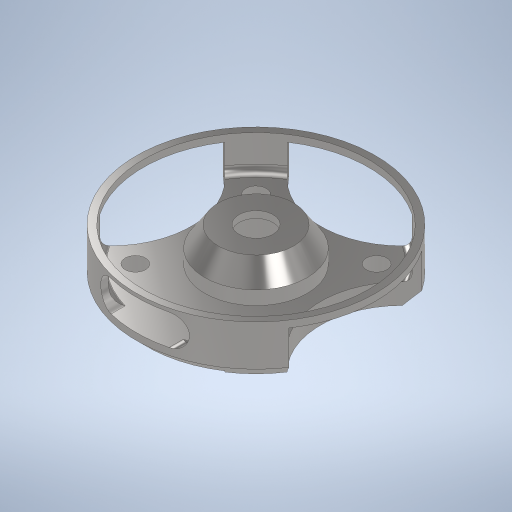
# Autodesk Inventor part: Base
Saved by Autodesk Inventor 2023.2 (Build 272271000, 271)
## iProperties
Created: 2023-03-04
Part Number: Base
Material: Stainless Steel
Document SubType Name: Modeling
Designer: Nathan Cai
Density: 8 g/cm^3
Appearance: Semi-Polished
Author: Nathan Cai
Autodesk Inventor part; units mm, degrees
ref_plane "YZ Plane" through (0, 0, 0) normal (1, 0, 0) x (0, 1, 0)
ref_plane "XZ Plane" through (0, 0, 0) normal (0, 1, 0) x (-1, 0, 0)
sketch "Sketch1" plane through (0, 0, 0) normal (0, 0, 1) x (1, 0, 0)
  line L0 (0, 0) -> (17.5, 0)
  line L1 (17.5, 0) -> (17.5, 8)
  line L2 (17.5, 8) -> (0, 8)
  line L3 (0, 8) -> (0, 0)
  line L4 (0, 8) -> (16.5, 8)
  line L5 (16.5, 8) -> (16.5, 3)
  line L6 (16.5, 3) -> (0, 3)
  line L7 (0, 3) -> (0, 8)
  line L8 (0, 3) -> (7.5, 3)
  line L9 (7.5, 3) -> (7.5, 5)
  line L10 (7.5, 5) -> (0, 5)
  line L11 (0, 5) -> (0, 3)
  line L12 (7.5, 5) -> (5.5, 8)
  line L13 (0, 8) -> (2.5, 8)
  line L14 (2.5, 8) -> (2.5, 0)
  line L15 (2.5, 0) -> (0, 0)
  line L16 (0, 0) -> (0, 8)
  point P0 (16.5, 5.5)
  dimension "d0" = 17.5
  dimension "d1" = 8
  dimension "d2" = 1
  dimension "d3" = 3
  dimension "d4" = 7.5
  dimension "d5" = 2
  dimension "d6" = 5.5
  dimension "d7" = 2.5
  constraints: 34 end point, 8 parallel, 4 horizontal, 4 perpendicular, 2 point on line, 1 midpoint
  measures "d0" distance of L2.end L1.end
  measures "d1" distance of L1.end L0.end
  measures "d2" distance from line of L1 point (16.5, 5.5)
  measures "d3" distance between parallel lines of L0 L6
  measures "d4" distance of L10.end L9.end
  measures "d5" distance of L9.end L8.end
  measures "d6" distance from line of L3 L12.end
  measures "d7" distance of L14.end L15.end
revolve "Revolution1" add sketch "Sketch1" angle 360 about axis through (0, 8, 0) along (0, -1, 0) contours L14 L6 L5 L2 L1 L0 | L14 L10 L9 L6 | L14 L2 L12 L10
chamfer "Chamfer1" distance 2 angle 45 1 edges at (-17.5, 0, 0)
fillet "Fillet1" radius 1 1 edges at (-16.5, 3, 0)
sketch "Sketch2" plane through (0, 0, 0) normal (0, -1, 0) x (1, 0, 0)
  circle A0 centre (0, 0) radius 12.5 construction
  line L0 (0, 12.5) -> (0, 0) construction
  circle A1 centre (0, 0) radius 2.5 projected
  circle A2 centre (0, 0) radius 15.5 projected
  circle A3 centre (0, 0) radius 15.5 projected
  line L1 (0, 0) -> (-8.8388, 8.8388) construction
  circle A4 centre (-8.8388, 8.8388) radius 1.5
  circle A5 centre (-8.8388, -8.8388) radius 1.5
  circle A6 centre (8.8388, -8.8388) radius 1.5
  circle A7 centre (8.8388, 8.8388) radius 1.5
  line L2 (-8.4184, 13.0146) -> (-13.0146, 8.4184) construction
  line L3 (8.4184, 13.0146) -> (13.0146, 8.4184) construction
  circle A8 centre (0, 0) radius 9.5 construction
  circle A9 centre (0, 21.433) radius 11.933
  circle A10 centre (-21.433, 0) radius 11.933
  circle A11 centre (0, -21.433) radius 11.933
  circle A12 centre (21.433, 0) radius 11.933
  circle A13 centre (0, 0) radius 5.5
  point P0 (-10.7165, 10.7165)
  point P1 (-8.4421, -12.9993)
  point P2 (8.4421, -12.9993)
  dimension "d13" = 25
  dimension "d15" = 45
  dimension "d16" = 3
  dimension "d19" = 360
  dimension "d21" = 6.5
  dimension "d22" = 19
  dimension "d25" = 360
  dimension "d27" = 11
  constraints: 11 centre point, 8 end point, 4 coincident, 4 point on circle, 2 line through centre, 2 symmetric about line, 1 midpoint, 1 point on line, 1 tangent, 1 vertical, 18 other
  measures "d13" diameter of A0
  measures "d15" angle of L0 L1
  measures "d16" diameter of A4
  measures "d21" distance of L2.start L2.end
  measures "d22" diameter of A8
  measures "d27" diameter of A13
extrude "Extrusion1" cut sketch "Sketch2" against normal blind 7 contours A1 | A2 A12 | A2 A12 | A11 A2 | A2 A11 | A10 A2 | A2 A10 | A4 | A5 | A6 | A7 | A13
extrude "Extrusion2" cut sketch "Sketch2" against normal blind 0.5 contours A9 A2 | A2 A9
ref_plane "Work Plane1" through (0, 0, 10) normal (0, 0, 1) x (1, 0, 0)
sketch "Sketch3" plane through (0, 0, 10) normal (0, 0, 1) x (1, 0, 0)
  line L0 (-17.5, 8) -> (17.5, 8) projected
  line L1 (0, 8) -> (0, 0) construction
  line L2 (-4.25, 5.25) -> (4.25, 5.25) construction
  line L3 (5.5, 0) -> (-5.5, 0) projected
  line L4 (-4.25, 3) -> (4.25, 3)
  line L5 (4.25, 7.5) -> (-4.25, 7.5)
  arc A0 (-4.25, 7.5) -> (-4.25, 3) centre (-4.25, 5.25) ccw
  arc A1 (4.25, 3) -> (4.25, 7.5) centre (4.25, 5.25) ccw
  line L6 (8.7938, 0.5) -> (-8.7938, 0.5) projected
  point P0 (0, 5.25)
  dimension "d33" = 2.5
  dimension "d34" = 2.25
  dimension "d35" = 8.5
  constraints: 10 end point, 4 point on circle, 4 tangent, 2 centre point, 2 midpoint, 2 parallel, 1 point on line, 1 vertical
  measures "d33" distance between parallel lines of L6 L4
  measures "d34" radius of A1
  measures "d35" distance of L2.start L2.end
extrude "Extrusion3" cut sketch "Sketch3" along normal through all
body "Solid1"
